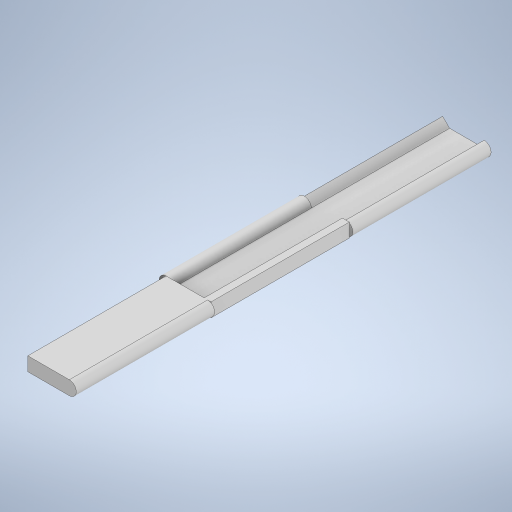
# Autodesk Inventor part: edges
Saved by Autodesk Inventor 2023.1 (Build 271208000, 208)
## iProperties
Created: 2022-09-07
Part Number: edges
Material: Generic
Document SubType Name: Modeling
Designer: swang
Density: 1 g/cm^3
Appearance: Default
Author: swang
## iProperties of the stored document edges_3DPrint.ipt
Created: 2022-09-07
Part Number: edges_3DPrint
Material: Generic
Document SubType Name: Modeling
Designer: swang
Density: 1 g/cm^3
Appearance: Default
Author: swang
Autodesk Inventor part; units mm, degrees
ref_plane "YZ Plane" through (0, 0, 0) normal (1, 0, 0) x (0, 1, 0)
ref_plane "XZ Plane" through (0, 0, 0) normal (0, 1, 0) x (-1, 0, 0)
ref_plane "XY Plane" through (0, 0, 0) normal (0, 0, 1) x (1, 0, 0)
sketch "Sketch1" plane through (0, 0, 0) normal (0, 0, 1) x (1, 0, 0)
  line L0 (0, 0) -> (30, 0)
  line L1 (30, 0) -> (30, 10)
  line L2 (30, 10) -> (0, 10)
  line L3 (0, 10) -> (0, 0)
  dimension "d0" = 30
  dimension "d1" = 10
  constraints: 8 end point, 2 parallel, 1 horizontal, 1 perpendicular
  measures "d0" distance of L1.end L2.end
  measures "d1" distance of L0.end L1.end
extrude "Extrusion1" add sketch "Sketch1" along normal blind 100
sketch "Sketch2" plane through (0, 0, 0) normal (0, 0, -1) x (-1, 0, 0)
  line L0 (0, 10) -> (0, 0) projected
  line L1 (-30, 10) -> (0, 10) projected
  arc A0 (0, 0) -> (-5, 5) centre (0, 5) ccw
  line L2 (-30, 0) -> (-30, 10) projected
  line L3 (-30, 5) -> (-5, 5)
  line L4 (0, 0) -> (-30, 0)
  line L5 (-30, 0) -> (-30, 5)
  constraints: 6 end point, 3 point on circle, 2 midpoint, 1 centre point, 1 horizontal, 1 parallel
extrude "Extrusion2" add sketch "Sketch2" along normal blind 100 contours A0 L0 | L0 L4 L2 L3 A0
sketch "Sketch3" plane through (0, 0, -100) normal (0, 0, -1) x (-1, 0, 0)
  line L0 (-30, 10) -> (0, 10) projected
  line L1 (0, 10) -> (-5, 5)
  arc A0 (0, 0) -> (-5, 5) centre (0, 5) ccw projected
  line L2 (0, 10) -> (5, 5)
  line L3 (-30, 0) -> (-30, 10) projected
  line L4 (-30, 5) -> (-5, 5)
  line L5 (5, 5) -> (5, 0)
  line L6 (5, 0) -> (-30, 0)
  line L7 (-30, 0) -> (-30, 5)
  constraints: 12 end point, 3 point on circle, 2 parallel, 2 perpendicular, 1 horizontal, 1 midpoint
extrude "Extrusion3" add sketch "Sketch3" along normal blind 100 contours L2 A0 L6 L3 L4 L1
sketch "Sketch4" plane through (0, 0, 100) normal (0, 0, 1) x (1, 0, 0)
  line L0 (30, 5) -> (5, 5) projected
  line L1 (30, 0) -> (30, 10) projected
  arc A0 (30, 0) -> (30, 10) centre (30, 5) ccw
  line L2 (30, 10) -> (30, 0)
  point P0 (0, 0)
  constraints: 2 end point, 2 point on circle, 1 centre point, 1 collinear, 1 point on line
extrude "Extrusion4" add sketch "Sketch4" against normal up to surface (100 mm away)
sketch "Sketch5" plane through (0, 0, 0) normal (0, 0, -1) x (-1, 0, 0)
  line L0 (-30, 10) -> (0, 10) projected
  line L1 (-32.5, 0) -> (-27.5, 0)
  line L2 (-27.5, 0) -> (-27.5, 10)
  line L3 (-27.5, 10) -> (-32.5, 10)
  line L4 (-32.5, 10) -> (-32.5, 0)
  line L5 (-30, 5) -> (-5, 5) projected
  line L6 (-32.5, 0) -> (-27.5, 10) construction
  line L7 (-27.5, 0) -> (-32.5, 10) construction
  point P0 (0, 0)
  dimension "d10" = 5
  constraints: 12 end point, 2 midpoint, 2 parallel, 1 horizontal, 1 perpendicular, 1 point on line
  measures "d10" distance of L2.end L3.end
extrude "Extrusion5" add sketch "Sketch5" along normal blind 100
sketch "Sketch6" plane through (0, 0, -200) normal (0, 0, -1) x (-1, 0, 0)
  line L0 (-5, 5) -> (-30, 5) projected
  arc A0 (-30, 10) -> (-30, 0) centre (-30, 5) ccw
  line L1 (-30, 10) -> (0, 10) projected
  line L2 (-30, 5) -> (-30, 0) projected
  line L3 (-30, 10) -> (-30, 0)
  point P0 (0, 0)
  constraints: 2 end point, 2 point on circle, 1 centre point, 1 collinear, 1 point on line, 1 tangent
extrude "Extrusion6" add sketch "Sketch6" against normal up to surface (100 mm away)
body "Solid1"
